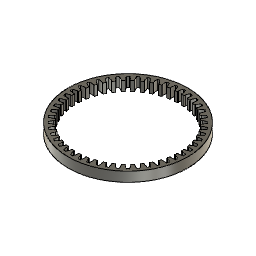
second_internal_gear_34.994mm_diameter v1 (Autodesk Fusion 360 design; units mm, degrees)
Autodesk Fusion 360 part; units mm, degrees
sketch "Sketch1" plane through (0, 0, 0) normal (0, 0, 1) x (1, 0, 0)
  spline S0 degree 5 poles (16.2535, -0.6223) (16.2536, -0.6223) (16.2537, -0.6223) (16.2539, -0.6223) (16.2541, -0.6223) (16.2546, -0.6223) (16.2551, -0.6224) (16.2556, -0.6224) (16.2562, -0.6224) (16.2569, -0.6224) (16.2576, -0.6224) (16.2584, -0.6224) (16.2593, -0.6224) (16.2602, -0.6224) (16.2612, -0.6224) (16.2622, -0.6224) (16.2633, -0.6225) (16.2644, -0.6225) (16.2656, -0.6225) (16.2669, -0.6225) (16.2682, -0.6224) (16.2696, -0.6224) (16.271, -0.6224) (16.2725, -0.6224) (16.2741, -0.6224) (16.2757, -0.6224) (16.2773, -0.6223) (16.279, -0.6223) (16.2808, -0.6223) (16.2826, -0.6222) (16.2844, -0.6222) (16.2864, -0.6222) (16.2883, -0.6221) (16.2903, -0.622) (16.2924, -0.622) (16.2945, -0.6219) (16.2967, -0.6218) (16.2989, -0.6218) (16.3012, -0.6217) (16.3035, -0.6216) (16.3059, -0.6215) (16.3083, -0.6214) (16.3108, -0.6213) (16.3133, -0.6211) (16.3159, -0.621) (16.3185, -0.6209) (16.3211, -0.6207) (16.3238, -0.6206) (16.3266, -0.6204) (16.3294, -0.6203) (16.3322, -0.6201) (16.3351, -0.6199) (16.3381, -0.6198) (16.3411, -0.6196) (16.3441, -0.6194) (16.3472, -0.6191) (16.3503, -0.6189) (16.3534, -0.6187) (16.3566, -0.6185) (16.3599, -0.6182) (16.3632, -0.618) (16.3665, -0.6177) (16.3699, -0.6174) (16.3733, -0.6171) (16.3768, -0.6168) (16.3803, -0.6165) (16.3839, -0.6162) (16.3874, -0.6159) (16.3911, -0.6156) (16.3947, -0.6152) (16.3985, -0.6149) (16.4022, -0.6145) (16.406, -0.6141) (16.4099, -0.6138) (16.4137, -0.6134) (16.4176, -0.613) (16.4216, -0.6125) (16.4256, -0.6121) (16.4296, -0.6117) (16.4337, -0.6112) (16.4378, -0.6108) (16.442, -0.6103) (16.4462, -0.6098) (16.4504, -0.6093) (16.4546, -0.6088) (16.4589, -0.6083) (16.4633, -0.6077) (16.4677, -0.6072) (16.4721, -0.6066) (16.4765, -0.6061) (16.481, -0.6055) (16.4855, -0.6049) (16.4901, -0.6043) (16.4947, -0.6037) (16.4993, -0.603) (16.504, -0.6024) (16.5087, -0.6017) (16.5134, -0.6011) (16.5182, -0.6004) (16.523, -0.5997) (16.5279, -0.599) (16.5328, -0.5983) (16.5377, -0.5975) (16.5426, -0.5968) (16.5476, -0.596) (16.5526, -0.5953) (16.5577, -0.5945) (16.5627, -0.5937) (16.5679, -0.5928) (16.573, -0.592) (16.5782, -0.5912) (16.5834, -0.5903) (16.5886, -0.5894) (16.5939, -0.5886) (16.5992, -0.5877) (16.6046, -0.5867) (16.61, -0.5858) (16.6154, -0.5849) (16.6208, -0.5839) (16.6263, -0.5829) (16.6318, -0.5819) (16.6373, -0.5809) (16.6429, -0.5799) (16.6485, -0.5789) (16.6541, -0.5779) (16.6598, -0.5768) (16.6655, -0.5757) (16.6712, -0.5746) (16.6769, -0.5735) (16.6827, -0.5724) (16.6885, -0.5713) (16.6943, -0.5701) (16.7002, -0.5689) (16.7061, -0.5678) (16.712, -0.5666) (16.718, -0.5653) (16.724, -0.5641) (16.73, -0.5629) (16.736, -0.5616) (16.7421, -0.5603) (16.7482, -0.559) (16.7543, -0.5577) (16.7605, -0.5564) (16.7667, -0.5551) (16.7729, -0.5537) (16.7791, -0.5523) (16.7854, -0.5509) (16.7917, -0.5495) (16.798, -0.5481) (16.8043, -0.5467) (16.8107, -0.5452) (16.8171, -0.5438) (16.8235, -0.5423) (16.83, -0.5408) (16.8365, -0.5392) (16.843, -0.5377) (16.8495, -0.5361) (16.8561, -0.5346) (16.8626, -0.533) (16.8693, -0.5314) (16.8759, -0.5298) (16.8826, -0.5281) (16.8892, -0.5265) (16.896, -0.5248) (16.9027, -0.5231) (16.9095, -0.5214) (16.9162, -0.5197) (16.9231, -0.5179) (16.9299, -0.5162) (16.9368, -0.5144) (16.9436, -0.5126) (16.9506, -0.5108) (16.9575, -0.509) (16.9645, -0.5071) (16.9714, -0.5053) (16.9784, -0.5034) (16.9855, -0.5015) (16.9925, -0.4996) (16.9996, -0.4977) (17.0067, -0.4957) (17.0138, -0.4937) (17.021, -0.4917) (17.0282, -0.4897) (17.0354, -0.4877) (17.0426, -0.4857) (17.0498, -0.4836) (17.0571, -0.4816) (17.0644, -0.4795) (17.0717, -0.4774) (17.079, -0.4752) (17.0864, -0.4731) (17.0937, -0.4709) (17.1011, -0.4687) (17.1085, -0.4665) (17.116, -0.4643) (17.1234, -0.4621) (17.1309, -0.4598) (17.1384, -0.4575) (17.146, -0.4552) (17.1535, -0.4529) (17.1611, -0.4506) (17.1687, -0.4483) (17.1763, -0.4459) (17.1839, -0.4435) (17.1916, -0.4411) (17.1992, -0.4387) (17.2069, -0.4362) (17.2146, -0.4338) (17.2224, -0.4313) (17.2301, -0.4288) (17.2379, -0.4263) (17.2457, -0.4237) (17.2535, -0.4212) (17.2614, -0.4186) (17.2692, -0.416) (17.2771, -0.4134) (17.285, -0.4108) (17.2929, -0.4081) (17.3008, -0.4055) (17.3088, -0.4028) (17.3167, -0.4001) (17.3247, -0.3973) (17.3327, -0.3946) (17.3408, -0.3918) (17.3488, -0.3891) (17.3569, -0.3863) (17.365, -0.3834) (17.3731, -0.3806) (17.3812, -0.3777) (17.3893, -0.3749) (17.3975, -0.372) (17.4057, -0.369) (17.4139, -0.3661) (17.4221, -0.3631) (17.4303, -0.3602) (17.4386, -0.3572) (17.4468, -0.3542) (17.4551, -0.3511) (17.4634, -0.3481) (17.4717, -0.345) (17.4801, -0.3419) (17.4867, -0.3394) (17.4918, -0.3375) (17.4951, -0.3363) (17.4968, -0.3357) knots 0 0 0 0 0 0 0.00416667 0.00833333 0.0125 0.01666667 0.02083333 0.025 0.02916667 0.03333333 0.0375 0.04166667 0.04583333 0.05 0.05416667 0.05833333 0.0625 0.06666667 0.07083333 0.075 0.07916667 0.08333333 0.0875 0.09166667 0.09583333 0.1 0.10416667 0.10833333 0.1125 0.11666667 0.12083333 0.125 0.12916667 0.13333333 0.1375 0.14166667 0.14583333 0.15 0.15416667 0.15833333 0.1625 0.16666667 0.17083333 0.175 0.17916667 0.18333333 0.1875 0.19166667 0.19583333 0.2 0.20416667 0.20833333 0.2125 0.21666667 0.22083333 0.225 0.22916667 0.23333333 0.2375 0.24166667 0.24583333 0.25 0.25416667 0.25833333 0.2625 0.26666667 0.27083333 0.275 0.27916667 0.28333333 0.2875 0.29166667 0.29583333 0.3 0.30416667 0.30833333 0.3125 0.31666667 0.32083333 0.325 0.32916667 0.33333333 0.3375 0.34166667 0.34583333 0.35 0.35416667 0.35833333 0.3625 0.36666667 0.37083333 0.375 0.37916667 0.38333333 0.3875 0.39166667 0.39583333 0.4 0.40416667 0.40833333 0.4125 0.41666667 0.42083333 0.425 0.42916667 0.43333333 0.4375 0.44166667 0.44583333 0.45 0.45416667 0.45833333 0.4625 0.46666667 0.47083333 0.475 0.47916667 0.48333333 0.4875 0.49166667 0.49583333 0.5 0.50416667 0.50833333 0.5125 0.51666667 0.52083333 0.525 0.52916667 0.53333333 0.5375 0.54166667 0.54583333 0.55 0.55416667 0.55833333 0.5625 0.56666667 0.57083333 0.575 0.57916667 0.58333333 0.5875 0.59166667 0.59583333 0.6 0.60416667 0.60833333 0.6125 0.61666667 0.62083333 0.625 0.62916667 0.63333333 0.6375 0.64166667 0.64583333 0.65 0.65416667 0.65833333 0.6625 0.66666667 0.67083333 0.675 0.67916667 0.68333333 0.6875 0.69166667 0.69583333 0.7 0.70416667 0.70833333 0.7125 0.71666667 0.72083333 0.725 0.72916667 0.73333333 0.7375 0.74166667 0.74583333 0.75 0.75416667 0.75833333 0.7625 0.76666667 0.77083333 0.775 0.77916667 0.78333333 0.7875 0.79166667 0.79583333 0.8 0.80416667 0.80833333 0.8125 0.81666667 0.82083333 0.825 0.82916667 0.83333333 0.8375 0.84166667 0.84583333 0.85 0.85416667 0.85833333 0.8625 0.86666667 0.87083333 0.875 0.87916667 0.88333333 0.8875 0.89166667 0.89583333 0.9 0.90416667 0.90833333 0.9125 0.91666667 0.92083333 0.925 0.92916667 0.93333333 0.9375 0.94166667 0.94583333 0.95 0.95416667 0.95833333 0.9625 0.96666667 0.97083333 0.975 0.97916667 0.98333333 0.9875 0.99166667 0.99583333 1 1 1 1 1 1
  spline S1 degree 5 poles (16.2535, 0.6223) (16.2536, 0.6223) (16.2537, 0.6223) (16.2539, 0.6223) (16.2541, 0.6223) (16.2546, 0.6223) (16.2551, 0.6224) (16.2556, 0.6224) (16.2562, 0.6224) (16.2569, 0.6224) (16.2576, 0.6224) (16.2584, 0.6224) (16.2593, 0.6224) (16.2602, 0.6224) (16.2612, 0.6224) (16.2622, 0.6224) (16.2633, 0.6225) (16.2644, 0.6225) (16.2656, 0.6225) (16.2669, 0.6225) (16.2682, 0.6224) (16.2696, 0.6224) (16.271, 0.6224) (16.2725, 0.6224) (16.2741, 0.6224) (16.2757, 0.6224) (16.2773, 0.6223) (16.279, 0.6223) (16.2808, 0.6223) (16.2826, 0.6222) (16.2844, 0.6222) (16.2864, 0.6222) (16.2883, 0.6221) (16.2903, 0.622) (16.2924, 0.622) (16.2945, 0.6219) (16.2967, 0.6218) (16.2989, 0.6218) (16.3012, 0.6217) (16.3035, 0.6216) (16.3059, 0.6215) (16.3083, 0.6214) (16.3108, 0.6213) (16.3133, 0.6211) (16.3159, 0.621) (16.3185, 0.6209) (16.3211, 0.6207) (16.3238, 0.6206) (16.3266, 0.6204) (16.3294, 0.6203) (16.3322, 0.6201) (16.3351, 0.6199) (16.3381, 0.6198) (16.3411, 0.6196) (16.3441, 0.6194) (16.3472, 0.6191) (16.3503, 0.6189) (16.3534, 0.6187) (16.3566, 0.6185) (16.3599, 0.6182) (16.3632, 0.618) (16.3665, 0.6177) (16.3699, 0.6174) (16.3733, 0.6171) (16.3768, 0.6168) (16.3803, 0.6165) (16.3839, 0.6162) (16.3874, 0.6159) (16.3911, 0.6156) (16.3947, 0.6152) (16.3985, 0.6149) (16.4022, 0.6145) (16.406, 0.6141) (16.4099, 0.6138) (16.4137, 0.6134) (16.4176, 0.613) (16.4216, 0.6125) (16.4256, 0.6121) (16.4296, 0.6117) (16.4337, 0.6112) (16.4378, 0.6108) (16.442, 0.6103) (16.4462, 0.6098) (16.4504, 0.6093) (16.4546, 0.6088) (16.4589, 0.6083) (16.4633, 0.6077) (16.4677, 0.6072) (16.4721, 0.6066) (16.4765, 0.6061) (16.481, 0.6055) (16.4855, 0.6049) (16.4901, 0.6043) (16.4947, 0.6037) (16.4993, 0.603) (16.504, 0.6024) (16.5087, 0.6017) (16.5134, 0.6011) (16.5182, 0.6004) (16.523, 0.5997) (16.5279, 0.599) (16.5328, 0.5983) (16.5377, 0.5975) (16.5426, 0.5968) (16.5476, 0.596) (16.5526, 0.5953) (16.5577, 0.5945) (16.5627, 0.5937) (16.5679, 0.5928) (16.573, 0.592) (16.5782, 0.5912) (16.5834, 0.5903) (16.5886, 0.5894) (16.5939, 0.5886) (16.5992, 0.5877) (16.6046, 0.5867) (16.61, 0.5858) (16.6154, 0.5849) (16.6208, 0.5839) (16.6263, 0.5829) (16.6318, 0.5819) (16.6373, 0.5809) (16.6429, 0.5799) (16.6485, 0.5789) (16.6541, 0.5779) (16.6598, 0.5768) (16.6655, 0.5757) (16.6712, 0.5746) (16.6769, 0.5735) (16.6827, 0.5724) (16.6885, 0.5713) (16.6943, 0.5701) (16.7002, 0.5689) (16.7061, 0.5678) (16.712, 0.5666) (16.718, 0.5653) (16.724, 0.5641) (16.73, 0.5629) (16.736, 0.5616) (16.7421, 0.5603) (16.7482, 0.559) (16.7543, 0.5577) (16.7605, 0.5564) (16.7667, 0.5551) (16.7729, 0.5537) (16.7791, 0.5523) (16.7854, 0.5509) (16.7917, 0.5495) (16.798, 0.5481) (16.8043, 0.5467) (16.8107, 0.5452) (16.8171, 0.5438) (16.8235, 0.5423) (16.83, 0.5408) (16.8365, 0.5392) (16.843, 0.5377) (16.8495, 0.5361) (16.8561, 0.5346) (16.8626, 0.533) (16.8693, 0.5314) (16.8759, 0.5298) (16.8826, 0.5281) (16.8892, 0.5265) (16.896, 0.5248) (16.9027, 0.5231) (16.9095, 0.5214) (16.9162, 0.5197) (16.9231, 0.5179) (16.9299, 0.5162) (16.9368, 0.5144) (16.9436, 0.5126) (16.9506, 0.5108) (16.9575, 0.509) (16.9645, 0.5071) (16.9714, 0.5053) (16.9784, 0.5034) (16.9855, 0.5015) (16.9925, 0.4996) (16.9996, 0.4977) (17.0067, 0.4957) (17.0138, 0.4937) (17.021, 0.4917) (17.0282, 0.4897) (17.0354, 0.4877) (17.0426, 0.4857) (17.0498, 0.4836) (17.0571, 0.4816) (17.0644, 0.4795) (17.0717, 0.4774) (17.079, 0.4752) (17.0864, 0.4731) (17.0937, 0.4709) (17.1011, 0.4687) (17.1085, 0.4665) (17.116, 0.4643) (17.1234, 0.4621) (17.1309, 0.4598) (17.1384, 0.4575) (17.146, 0.4552) (17.1535, 0.4529) (17.1611, 0.4506) (17.1687, 0.4483) (17.1763, 0.4459) (17.1839, 0.4435) (17.1916, 0.4411) (17.1992, 0.4387) (17.2069, 0.4362) (17.2146, 0.4338) (17.2224, 0.4313) (17.2301, 0.4288) (17.2379, 0.4263) (17.2457, 0.4237) (17.2535, 0.4212) (17.2614, 0.4186) (17.2692, 0.416) (17.2771, 0.4134) (17.285, 0.4108) (17.2929, 0.4081) (17.3008, 0.4055) (17.3088, 0.4028) (17.3167, 0.4001) (17.3247, 0.3973) (17.3327, 0.3946) (17.3408, 0.3918) (17.3488, 0.3891) (17.3569, 0.3863) (17.365, 0.3834) (17.3731, 0.3806) (17.3812, 0.3777) (17.3893, 0.3749) (17.3975, 0.372) (17.4057, 0.369) (17.4139, 0.3661) (17.4221, 0.3631) (17.4303, 0.3602) (17.4386, 0.3572) (17.4468, 0.3542) (17.4551, 0.3511) (17.4634, 0.3481) (17.4717, 0.345) (17.4801, 0.3419) (17.4867, 0.3394) (17.4918, 0.3375) (17.4951, 0.3363) (17.4968, 0.3357) knots 0 0 0 0 0 0 0.00416667 0.00833333 0.0125 0.01666667 0.02083333 0.025 0.02916667 0.03333333 0.0375 0.04166667 0.04583333 0.05 0.05416667 0.05833333 0.0625 0.06666667 0.07083333 0.075 0.07916667 0.08333333 0.0875 0.09166667 0.09583333 0.1 0.10416667 0.10833333 0.1125 0.11666667 0.12083333 0.125 0.12916667 0.13333333 0.1375 0.14166667 0.14583333 0.15 0.15416667 0.15833333 0.1625 0.16666667 0.17083333 0.175 0.17916667 0.18333333 0.1875 0.19166667 0.19583333 0.2 0.20416667 0.20833333 0.2125 0.21666667 0.22083333 0.225 0.22916667 0.23333333 0.2375 0.24166667 0.24583333 0.25 0.25416667 0.25833333 0.2625 0.26666667 0.27083333 0.275 0.27916667 0.28333333 0.2875 0.29166667 0.29583333 0.3 0.30416667 0.30833333 0.3125 0.31666667 0.32083333 0.325 0.32916667 0.33333333 0.3375 0.34166667 0.34583333 0.35 0.35416667 0.35833333 0.3625 0.36666667 0.37083333 0.375 0.37916667 0.38333333 0.3875 0.39166667 0.39583333 0.4 0.40416667 0.40833333 0.4125 0.41666667 0.42083333 0.425 0.42916667 0.43333333 0.4375 0.44166667 0.44583333 0.45 0.45416667 0.45833333 0.4625 0.46666667 0.47083333 0.475 0.47916667 0.48333333 0.4875 0.49166667 0.49583333 0.5 0.50416667 0.50833333 0.5125 0.51666667 0.52083333 0.525 0.52916667 0.53333333 0.5375 0.54166667 0.54583333 0.55 0.55416667 0.55833333 0.5625 0.56666667 0.57083333 0.575 0.57916667 0.58333333 0.5875 0.59166667 0.59583333 0.6 0.60416667 0.60833333 0.6125 0.61666667 0.62083333 0.625 0.62916667 0.63333333 0.6375 0.64166667 0.64583333 0.65 0.65416667 0.65833333 0.6625 0.66666667 0.67083333 0.675 0.67916667 0.68333333 0.6875 0.69166667 0.69583333 0.7 0.70416667 0.70833333 0.7125 0.71666667 0.72083333 0.725 0.72916667 0.73333333 0.7375 0.74166667 0.74583333 0.75 0.75416667 0.75833333 0.7625 0.76666667 0.77083333 0.775 0.77916667 0.78333333 0.7875 0.79166667 0.79583333 0.8 0.80416667 0.80833333 0.8125 0.81666667 0.82083333 0.825 0.82916667 0.83333333 0.8375 0.84166667 0.84583333 0.85 0.85416667 0.85833333 0.8625 0.86666667 0.87083333 0.875 0.87916667 0.88333333 0.8875 0.89166667 0.89583333 0.9 0.90416667 0.90833333 0.9125 0.91666667 0.92083333 0.925 0.92916667 0.93333333 0.9375 0.94166667 0.94583333 0.95 0.95416667 0.95833333 0.9625 0.96666667 0.97083333 0.975 0.97916667 0.98333333 0.9875 0.99166667 0.99583333 1 1 1 1 1 1
  spline S2 degree 5 poles (16.253, -0.6223) (16.253, -0.6223) (16.253, -0.6223) (16.2531, -0.6223) (16.2532, -0.6223) (16.2533, -0.6223) (16.2534, -0.6223) (16.2534, -0.6223) (16.2535, -0.6223) (16.2535, -0.6223) knots 0 0 0 0 0 0 0.2 0.4 0.6 0.8 1 1 1 1 1 1
  spline S3 degree 5 poles (16.253, 0.6223) (16.253, 0.6223) (16.253, 0.6223) (16.2531, 0.6223) (16.2532, 0.6223) (16.2533, 0.6223) (16.2534, 0.6223) (16.2534, 0.6223) (16.2535, 0.6223) (16.2535, 0.6223) knots 0 0 0 0 0 0 0.2 0.4 0.6 0.8 1 1 1 1 1 1
  line L0 (0, 0) -> (16.253, -0.6223)
  line L1 (0, 0) -> (16.253, 0.6223)
  arc A0 (17.4968, -0.3357) -> (17.4968, 0.3357) centre (0, 0) ccw
  point P0 (16.2551, -0.6224)
  point P1 (16.2578, -0.6224)
  point P2 (16.2615, -0.6224)
  point P3 (16.2663, -0.6225)
  point P4 (16.2722, -0.6224)
  point P5 (16.2791, -0.6223)
  point P6 (16.2871, -0.6221)
  point P7 (16.2962, -0.6219)
  point P8 (16.3063, -0.6215)
  point P9 (16.3176, -0.6209)
  point P10 (16.3298, -0.6203)
  point P11 (16.3431, -0.6194)
  point P12 (16.3575, -0.6184)
  point P13 (16.373, -0.6172)
  point P14 (16.3894, -0.6157)
  point P15 (16.407, -0.614)
  point P16 (16.4256, -0.6121)
  point P17 (16.4452, -0.6099)
  point P18 (16.4659, -0.6074)
  point P19 (16.4876, -0.6046)
  point P20 (16.5103, -0.6015)
  point P21 (16.5341, -0.5981)
  point P22 (16.5589, -0.5943)
  point P23 (16.5848, -0.5901)
  point P24 (16.6116, -0.5855)
  point P25 (16.6395, -0.5806)
  point P26 (16.6683, -0.5752)
  point P27 (16.6982, -0.5693)
  point P28 (16.7291, -0.5631)
  point P29 (16.7609, -0.5563)
  point P30 (16.7938, -0.5491)
  point P31 (16.8276, -0.5413)
  point P32 (16.8624, -0.533)
  point P33 (16.8982, -0.5242)
  point P34 (16.9349, -0.5149)
  point P35 (16.9726, -0.505)
  point P36 (17.0113, -0.4944)
  point P37 (17.0508, -0.4833)
  point P38 (17.0914, -0.4716)
  point P39 (17.1328, -0.4592)
  point P40 (17.1752, -0.4462)
  point P41 (17.2185, -0.4325)
  point P42 (17.2626, -0.4182)
  point P43 (17.3077, -0.4031)
  point P44 (17.3537, -0.3874)
  point P45 (17.4005, -0.3709)
  point P46 (17.4482, -0.3536)
  point P47 (16.2551, 0.6224)
  point P48 (16.2578, 0.6224)
  point P49 (16.2615, 0.6224)
  point P50 (16.2663, 0.6225)
  point P51 (16.2722, 0.6224)
  point P52 (16.2791, 0.6223)
  point P53 (16.2871, 0.6221)
  point P54 (16.2962, 0.6219)
  point P55 (16.3063, 0.6215)
  point P56 (16.3176, 0.6209)
  point P57 (16.3298, 0.6203)
  point P58 (16.3431, 0.6194)
  point P59 (16.3575, 0.6184)
  point P60 (16.373, 0.6172)
  point P61 (16.3894, 0.6157)
  point P62 (16.407, 0.614)
  point P63 (16.4256, 0.6121)
  point P64 (16.4452, 0.6099)
  point P65 (16.4659, 0.6074)
  point P66 (16.4876, 0.6046)
  point P67 (16.5103, 0.6015)
  point P68 (16.5341, 0.5981)
  point P69 (16.5589, 0.5943)
  point P70 (16.5848, 0.5901)
  point P71 (16.6116, 0.5855)
  point P72 (16.6395, 0.5806)
  point P73 (16.6683, 0.5752)
  point P74 (16.6982, 0.5693)
  point P75 (16.7291, 0.5631)
  point P76 (16.7609, 0.5563)
  point P77 (16.7938, 0.5491)
  point P78 (16.8276, 0.5413)
  point P79 (16.8624, 0.533)
  point P80 (16.8982, 0.5242)
  point P81 (16.9349, 0.5149)
  point P82 (16.9726, 0.505)
  point P83 (17.0113, 0.4944)
  point P84 (17.0508, 0.4833)
  point P85 (17.0914, 0.4716)
  point P86 (17.1328, 0.4592)
  point P87 (17.1752, 0.4462)
  point P88 (17.2185, 0.4325)
  point P89 (17.2626, 0.4182)
  point P90 (17.3077, 0.4031)
  point P91 (17.3537, 0.3874)
  point P92 (17.4005, 0.3709)
  point P93 (17.4482, 0.3536)
sketch "Sketch2" plane through (0, 0, 0) normal (0, 0, 1) x (1, 0, 0)
  circle A0 centre (0, 0) radius 18.5
  circle A1 centre (0, 0) radius 15.925
  circle A2 centre (0, 0) radius 15.925
extrude "Extrude1" add sketch "Sketch2" along normal blind 3
extrude "Extrude2" cut sketch "Sketch1" along normal blind 3
pattern_circular "C-Pattern1" count 48 over 360 about axis through (0, 0, 1.75) along (0, 0, 1) of "Extrude2"
sketch "Sketch3" plane through (0, 0, 0) normal (0, 0, 1) x (1, 0, 0)
  line L0 (0, 0) -> (48.7031, 0) construction
  line L1 (48.7031, 0) -> (48.7031, 3) construction
  line L2 (48.7031, 3) -> (0, 3) construction
  line L3 (0, 3) -> (0, 0) construction
  constraint perpendicular L0 L1
  constraint parallel L0 L2
  constraint parallel L1 L3
